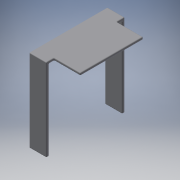
# Autodesk Inventor part: Footboard - feet protect holder
Saved by Autodesk Inventor 2018 (Build 220112000, 112)
## iProperties
Created: 2018-08-10
Part Number: Footboard - feet protect holder
Material: Generic
Document SubType Name: Modeling
Designer: ruben
Density: 1 g/cm^3
Sheet Metal Rule: Default_mm
Appearance: Default
Author: ruben
Autodesk Inventor part; units mm, degrees
ref_plane "YZ Plane" through (0, 0, 0) normal (1, 0, 0) x (0, 1, 0)
ref_plane "XZ Plane" through (0, 0, 0) normal (0, 1, 0) x (-1, 0, 0)
ref_plane "XY Plane" through (0, 0, 0) normal (0, 0, 1) x (1, 0, 0)
sketch "Sketch3" plane through (0, 0, 0) normal (0, 0, 1) x (1, 0, 0)
  line L0 (0, -66.5) -> (0, 66.5) projected
  line L1 (-63, 0) -> (63, 0) projected
  line L2 (-45, -47.5) -> (-42, -47.5)
  line L3 (-42, -47.5) -> (-42, 44.5)
  line L4 (-42, 44.5) -> (42, 44.5)
  line L5 (42, 44.5) -> (42, -47.5)
  line L6 (42, -47.5) -> (45, -47.5)
  line L7 (45, -47.5) -> (45, 47.5)
  line L8 (45, 47.5) -> (-45, 47.5)
  line L9 (-45, 47.5) -> (-45, -47.5)
  line L10 (-36, 47.5) -> (-36, 44.5)
  line L11 (36, 47.5) -> (36, 44.5)
  point P0 (0, 0)
  dimension "d0" = 3
  dimension "d2" = 3
  dimension "d4" = 95
  dimension "d5" = 95
  dimension "d6" = 90
  dimension "d9" = 72
  constraints: 20 end point, 9 perpendicular, 4 point on line, 1 horizontal, 4 other
  measures "d0" distance of L2.start L2.end
  measures "d2" distance between parallel lines of L4 L8
  measures "d4" distance between parallel lines of L2 L8
  measures "d5" distance between parallel lines of L6 L8
  measures "d6" distance between parallel lines of L7 L9
  measures "d9" distance between parallel lines of L11 L10
extrude "Extrusion1" add sketch "Sketch3" against normal blind 20 contours L4 L10 L8 L0 | L0 L8 L11 L4 | L3 L2 L9 L1 | L1 L9 L8 L10 L4 L3 | L5 L4 L11 L8 L7 L1 | L1 L7 L6 L5
extrude "Extrusion2" add sketch "Sketch3" along normal blind 30 contours L4 L10 L8 L0 | L0 L8 L11 L4
fillet "Fillet1" radius 1 30 edges at (-45, 0, 0) (-42, -1.5, 0) (-42, -1.5, -20) (-45, 0, -20) (0, 47.5, -20) (0, 44.5, -20) (-45, 47.5, -10) (-40.5, 47.5, 0) (-39, 44.5, 0) (-36, 44.5, 15) (0, 44.5, 30) (36, 46, 30) (36, 44.5, 15) (-36, 46, 30) (36, 46, 0) (-36, 46, 0) (45, 0, 0) (39, 44.5, 0) (42, -1.5, 0) (45, 0, -20) (42, -1.5, -20) (42, -47.5, -10) (45, -47.5, -10) (-42, -47.5, -10) (-45, -47.5, -10) (45, 47.5, -10) (40.5, 47.5, 0) (-36, 47.5, 15) (0, 47.5, 30) (36, 47.5, 15)
fillet "Fillet1" radius 1 4 edges at (-36, 46, 0) (36, 46, 0) (-42, 44.5, -10) (42, 44.5, -10)
fillet "Fillet1" radius 1 32 edges at (-45, 47.5, -10) (-45, -47.5, -10) (-45, 0, 0) (-45, 0, -20) (45, 47.5, -10) (0, 47.5, -20) (-40.5, 47.5, 0) (-36, 47.5, 15) (0, 47.5, 30) (36, 47.5, 15) (40.5, 47.5, 0) (-42, -47.5, -10) (-43.5, -47.5, 0) (-43.5, -47.5, -20) (-39, 44.5, 0) (-42, -1.5, 0) (45, 0, -20) (43.5, -47.5, -20) (42, -1.5, -20) (0, 44.5, -20) (-42, -1.5, -20) (45, -47.5, -10) (45, 0, 0) (43.5, -47.5, 0) (42, -1.5, 0) (39, 44.5, 0) (-36, 44.5, 15) (-36, 46, 30) (36, 44.5, 15) (0, 44.5, 30) (42, -47.5, -10) (36, 46, 30)
equation "\"d2\" = d0"
equation "\"d5\" = d4"
equation "\"BendRadius\" = Thickness"
equation "\"BendReliefWidth\" = Thickness"
equation "\"BendReliefDepth\" = 0.5 * Thickness"
equation "\"CornerReliefSize\" = 4 * Thickness"
equation "\"MinimumRemnant\" = 2 * Thickness"
equation "\"TransitionRadius\" = BendRadius"
equation "\"JacobiRadiusSize\" = BendRadius"
equation "\"GapSize\" = Thickness"
equation "\"Thickness\" = 0.5"
body "Solid1"
